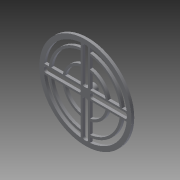
# Autodesk Inventor part: Scanning Disk
Saved by Autodesk Inventor 2015 (Build 190159000, 159)
## iProperties
Created: 2016-05-28
Part Number: Scanning Disk
Material: Generic
Document SubType Name: Modeling
Designer: Toby
Density: 1 g/cm^3
Appearance: Default
Author: Toby
Autodesk Inventor part; units mm, degrees
ref_plane "YZ Plane" through (0, 0, 0) normal (1, 0, 0) x (0, 1, 0)
ref_plane "XZ Plane" through (0, 0, 0) normal (0, 1, 0) x (-1, 0, 0)
ref_plane "XY Plane" through (0, 0, 0) normal (0, 0, 1) x (1, 0, 0)
sketch "Sketch1" plane through (0, 0, 0) normal (0, 1, 0) x (-1, 0, 0)
  circle A0 centre (0, 0) radius 50
  circle A1 centre (0, 0) radius 45
  line L0 (5, 48.7261) -> (-5, 48.7261)
  line L1 (-5, 48.7261) -> (-5, -48.4617)
  line L2 (-5, -48.4617) -> (5, -48.4617)
  line L3 (5, -48.4617) -> (5, 48.7261)
  line L4 (48.4415, 5) -> (-48.0304, 5)
  line L5 (-48.0304, 5) -> (-48.0304, -5)
  line L6 (-48.0304, -5) -> (48.4415, -5)
  line L7 (48.4415, -5) -> (48.4415, 5)
  dimension "d0" = 100
  dimension "d1" = 90
  dimension "d2" = 5
  dimension "d3" = 5
  dimension "d4" = 5
  dimension "d5" = 5
  constraints: 16 end point, 4 parallel, 2 centre point, 2 coincident, 2 horizontal, 2 perpendicular
  measures "d0" diameter of A0
  measures "d1" diameter of A1
  measures "d2" distance from line of point (0, 0) L4
  measures "d3" distance from line of point (0, 0) L6
  measures "d4" distance from line of point (0, 0) L1
  measures "d5" distance from line of point (0, 0) L3
extrude "Extrusion1" add sketch "Sketch1" along normal blind 3 contours A0 | A1 L6 L3 L4 | A1 L4 L7 L6 | L3 L4 L1 A1 | A1 L1 L0 L3 | L3 L6 L1 L4 | L3 L2 L1 A1 | A1 L1 L6 L3 | L1 L6 A1 L4 | A1 L6 L5 L4
sketch "Sketch2" plane through (0, 3, 0) normal (0, 1, 0) x (1, 0, 0)
  circle A0 centre (0, 0) radius 40
  circle A1 centre (0, 0) radius 37.5
  circle A2 centre (0, 0) radius 25
  circle A3 centre (0, 0) radius 22.5
  dimension "d8" = 80
  dimension "d9" = 75
  dimension "d10" = 50
  dimension "d11" = 45
  constraints: 4 centre point, 4 coincident
  measures "d8" diameter of A0
  measures "d9" diameter of A1
  measures "d10" diameter of A2
  measures "d11" diameter of A3
extrude "Extrusion2" add sketch "Sketch2" against normal blind 3
sketch "Sketch3" plane through (0, 3, 0) normal (0, 1, 0) x (1, 0, 0)
  circle A0 centre (0, 0) radius 4.5
  line L0 (-1.51, -3.1) -> (1.69, -3.1)
  line L1 (1.69, -3.1) -> (1.69, 3.1)
  line L2 (1.69, 3.1) -> (-1.51, 3.1)
  line L3 (-1.51, 3.1) -> (-1.51, -3.1)
  dimension "d14" = 9
  dimension "d15" = 6.2
  dimension "d16" = 3.2
  dimension "d17" = 1.51
  dimension "d18" = 3.1
  constraints: 8 end point, 2 parallel, 1 centre point, 1 coincident, 1 horizontal, 1 perpendicular
  measures "d14" diameter of A0
  measures "d15" distance of L2.end L0.start
  measures "d16" distance of L0.start L0.end
  measures "d17" distance from line of point (0, 0) L3
  measures "d18" distance from line of point (0, 0) L0
extrude "Extrusion3" add sketch "Sketch3" along normal blind 7
sketch "Sketch4" plane through (0, 3, 0) normal (0, 1, 0) x (1, 0, 0)
  point P0 (0, 0)
sketch "Sketch5" plane through (0, 0, 0) normal (0, -1, 0) x (1, 0, 0)
  line L0 (45, 3) -> (-45, 3)
  line L1 (-45, 3) -> (-45, -3)
  line L2 (-45, -3) -> (45, -3)
  line L3 (45, -3) -> (45, 3)
  line L4 (3, 45) -> (-3, 45)
  line L5 (-3, 45) -> (-3, -45)
  line L6 (-3, -45) -> (3, -45)
  line L7 (3, -45) -> (3, 45)
  point P0 (0, 0)
  dimension "d21" = 90
  dimension "d22" = 90
  dimension "d23" = 45
  dimension "d24" = 45
  dimension "d25" = 3
  dimension "d26" = 3
  dimension "d27" = 3
  dimension "d28" = 3
  constraints: 16 end point, 4 parallel, 2 horizontal, 2 perpendicular
  measures "d21" distance of L6.end L4.start
  measures "d22" distance of L0.start L0.end
  measures "d23" distance from line of point (0, 0) L3
  measures "d24" distance from line of point (0, 0) L4
  measures "d25" distance from line of point (0, 0) L7
  measures "d26" distance from line of L5 point (0, 0)
  measures "d27" distance from line of point (0, 0) L0
  measures "d28" distance from line of point (0, 0) L2
extrude "Extrusion4" cut sketch "Sketch5" against normal blind 3
sketch "Sketch6" plane through (0, 0, 0) normal (0, -1, 0) x (1, 0, 0)
  line L0 (5.0041, 4.9106) -> (-5, 4.9106)
  line L1 (-5, 4.9106) -> (-5, -5)
  line L2 (-5, -5) -> (5.0041, -5)
  line L3 (5.0041, -5) -> (5.0041, 4.9106)
  point P0 (0, 0)
  constraints: 8 end point, 2 parallel, 1 horizontal, 1 perpendicular
extrude "Extrusion5" add sketch "Sketch6" against normal blind 3
fillet "Fillet1" radius 2 8 edges at (3, 1.5, 4.9106) (-3, 1.5, 4.9106) (-5, 1.5, 3) (-5, 1.5, -3) (-3, 1.5, -5) (3, 1.5, -5) (5.0041, 1.5, -3) (5.0041, 1.5, 3)
fillet "Fillet2" radius 2 8 edges at (45, 1.5, 3) (45, 1.5, -3) (3, 1.5, 45) (-3, 1.5, 45) (-45, 1.5, 3) (-45, 1.5, -3) (-3, 1.5, -45) (3, 1.5, -45)
body "Solid1"
